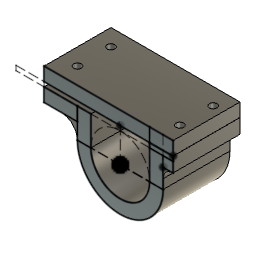
floorcowl_topfloor_edge v11 (Autodesk Fusion 360 design; units mm, degrees)
Autodesk Fusion 360 part; units mm, degrees
note: some values were not read from the file. Chosen so that the rebuilt part matches the saved one: which bodies a step acts on; which face or edge a step refers to.
sketch "Sketch1" plane through (0, 0, 0) normal (0, 1, 0) x (1, 0, 0)
  circle A0 centre (0, 0) radius 11.176 construction
  line L0 (0, 0) -> (0, -11.176) construction
  line L1 (0, -11.176) -> (0, -12.9286) construction
  line L2 (0, 0) -> (11.176, 0) construction
  line L3 (11.176, 0) -> (11.176, -11.176) construction
  line L4 (11.176, -11.176) -> (-39.624, -11.176) construction
  line L5 (-39.624, -11.176) -> (-39.624, -12.9286) construction
  line L6 (-39.624, -12.9286) -> (11.176, -12.9286) construction
  line L7 (11.176, -12.9286) -> (11.176, -11.176) construction
  line L8 (11.176, -12.9286) -> (-28.956, -12.9286)
  line L9 (-28.956, -12.9286) -> (-28.956, -18.0086)
  line L10 (-28.956, -18.0086) -> (11.176, -18.0086)
  line L11 (11.176, -18.0086) -> (11.176, -12.9286) construction
  line L12 (11.176, -18.0086) -> (16.256, -18.0086)
  line L13 (16.256, -18.0086) -> (16.256, 0)
  line L14 (16.256, 0) -> (11.176, 0)
  line L15 (11.176, 0) -> (11.176, -18.0086)
  arc A1 (16.256, 0) -> (-16.256, 0) centre (0, 0) ccw
  line L16 (0, 0) -> (16.256, 0) construction
  line L17 (0, 0) -> (-16.256, 0) construction
  arc A2 (11.176, 0) -> (-11.176, 0) centre (0, 0) ccw
  line L18 (0, 0) -> (11.176, 0) construction
  line L19 (0, 0) -> (-11.176, 0) construction
  line L20 (-11.176, 0) -> (-16.256, 0)
  line L21 (-16.256, 0) -> (-16.256, -11.176)
  line L22 (-16.256, -11.176) -> (-11.176, -11.176)
  line L23 (-11.176, -11.176) -> (-11.176, 0)
  line L24 (-16.256, -11.176) -> (-28.956, -11.176)
  line L25 (-28.956, -11.176) -> (-28.956, -6.096)
  line L26 (-28.956, -6.096) -> (-16.256, -6.096)
  line L27 (-16.256, -6.096) -> (-16.256, -11.176)
  line L28 (-28.956, -11.176) -> (-28.956, -12.9286) construction
  line L29 (16.256, -18.0086) -> (20.066, -18.0086)
  line L30 (20.066, -18.0086) -> (20.066, -12.9286)
  line L31 (11.176, -11.176) -> (16.256, -11.176)
  line L32 (16.256, -12.9286) -> (11.176, -12.9286) construction
  line L33 (20.066, -12.9286) -> (20.066, -11.176) construction
  line L34 (20.066, -11.176) -> (16.256, -11.176)
  line L35 (16.256, 0) -> (16.256, -11.176)
  line L36 (20.066, -11.176) -> (20.066, -7.366)
  line L37 (20.066, -7.366) -> (16.256, -7.366)
  line L38 (20.066, -12.9286) -> (11.176, -12.9286)
  line L39 (20.066, -11.176) -> (20.066, -12.8778)
  line L40 (20.066, -12.8778) -> (11.176, -12.8778)
  line L41 (11.176, -12.8778) -> (11.176, -11.176)
  line L42 (11.176, -11.176) -> (20.066, -11.176) construction
  line L43 (20.066, -11.176) -> (20.066, -12.8778)
  dimension "d1" = 22.352
  dimension "d2" = 1.7526
  dimension "d4" = 90
  dimension "d5" = 11.176
  dimension "d6" = 50.8
  dimension "d7" = 1.7526
  dimension "d9" = 5.08
  dimension "d10" = 5.08
  dimension "d11" = 18.0086
  dimension "d12" = 180
  dimension "d13" = 180
  dimension "d14" = 5.08
  dimension "d15" = 11.176
  dimension "d16" = 12.7
  dimension "d17" = 5.08
  dimension "d33" = 1.7526
  dimension "d42" = 3.81
  dimension "d43" = 5.08
  dimension "d44" = 1.7526
  dimension "d45" = 3.81
  dimension "d46" = 3.81
  dimension "d47" = 3.81
  dimension "d57" = 1.7018
  constraint coincident A0.centre L0.start
  constraint coincident A0 L0.end
  constraint vertical L0
  constraint parallel L0 L1
  constraint coincident A0 L2.end
  constraint perpendicular L0 L2
  constraint horizontal L4
  constraint vertical L5
  constraint horizontal L6
  constraint vertical L7
  constraint horizontal L8
  constraint vertical L9
  constraint horizontal L10
  constraint vertical L11
  constraint horizontal L12
  constraint vertical L13
  constraint horizontal L14
  constraint vertical L15
  constraint horizontal L20
  constraint vertical L21
  constraint horizontal L22
  constraint vertical L23
  constraint horizontal L24
  constraint vertical L25
  constraint horizontal L26
  constraint vertical L27
  constraint vertical L28
  constraint perpendicular L13 L29
  constraint perpendicular L29 L30
  constraint coincident L13 L32.start
  constraint coincident L13 L31.end
  constraint perpendicular L13 L31
  constraint horizontal L34
  constraint vertical L33
  constraint perpendicular L34 L36
  constraint perpendicular L13 L37
  constraint horizontal L32
  constraint perpendicular L34 L39
  constraint horizontal L40
  constraint vertical L41
  constraint horizontal L42
  constraint vertical L43
  measures "d1" diameter of A0
  measures "d2" distance of L0.end L1.end
  measures "d4" angle of L2 L3
  measures "d5" distance of L2.end L3.end
  measures "d6" distance of L3.end L4.end
  measures "d7" distance of L3.end L6.end
  measures "d9" distance of L6.end L10.end
  measures "d10" distance of L10.end L12.end
  measures "d11" distance of L12.end L13.end
  measures "d12" angle of L16 L17
  measures "d13" angle of L18 L19
  measures "d14" distance of A2.end A1.end
  measures "d15" distance of A2.end L22.end
  measures "d16" distance of L21.end L24.end
  measures "d17" distance of L21.end L26.end
  measures "d33" distance of L24.end L8.end
  measures "d42" distance of L12.end L29.end
  measures "d43" distance of L29.end L30.end
  measures "d44" distance of L30.end L33.end
  measures "d45" distance of L31.end L33.end
  measures "d46" distance of L33.end L36.end
  measures "d47" distance of L36.end L37.end
  measures "d57" distance of L33.end L39.end
extrude "Extrude1" add sketch "Sketch1" along normal blind 25.4 contours L8 L9 L10 L15 | L13 L14 L15 L31 L35 | L14 A1 A2 L20 | L20 L21 L22 L23 L27 | L21 L24 L25 L26 L27 makes body 1 at (-15.5787, 8.4667, 18.0086) makes body 2 at (-12.4528, 8.4667, -10.4492)
extrude "Extrude3" add sketch "Sketch1" along normal blind 25.4 contours L13 L15 L31 L40 L41 | L13 L34 L39 L40 L43 bodies 2
fillet "Fillet1" radius 6.35 1 edges at (-16.256, 12.7, 6.096) on bodies 2
sketch "Sketch4" plane through (0, 0, 18.0086) normal (0, 0, 1) x (-1, 0, 0)
  line L0 (28.956, 0) -> (-11.176, 0)
  line L1 (-11.176, -25.4) -> (28.956, -25.4)
  line L2 (28.956, -25.4) -> (28.956, 0)
  line L3 (28.956, -25.4) -> (16.256, -25.4)
  line L4 (16.256, -25.4) -> (16.256, 0)
  line L5 (16.256, 0) -> (28.956, 0)
  line L6 (28.956, 0) -> (28.956, -25.4)
  line L7 (28.956, -12.7) -> (16.256, -12.7)
  line L8 (22.606, -25.4) -> (22.606, 0)
  line L9 (-11.176, 0) -> (-11.176, -25.4)
  line L10 (-11.176, -25.4) -> (-16.256, -25.4) construction
  line L11 (-16.256, -25.4) -> (-16.256, 0) construction
  line L12 (-16.256, 0) -> (-11.176, 0) construction
  line L13 (16.256, -12.7) -> (-16.256, -12.7)
  point P0 (22.606, -19.05)
  point P1 (22.606, -6.35)
  point P2 (-16.256, -19.05)
  point P3 (-16.256, -6.35)
  dimension "d34" = 12.7
  dimension "d35" = 25.4
  dimension "d36" = 6.35
  dimension "d52" = 5.08
  dimension "d55" = 6.35
  dimension "d56" = 6.35
  constraint horizontal L3
  constraint vertical L4
  constraint horizontal L5
  constraint vertical L6
  constraint coincident L1.end L2.start
  constraint midpoint L2 L7.start
  constraint midpoint L4 L7.end
  constraint midpoint L3 L8.start
  constraint midpoint L5 L8.end
  constraint coincident L8 P0
  constraint symmetric L7 P0 P1
  constraint coincident L1.start L9.end
  constraint perpendicular L9 L10
  constraint perpendicular L10 L11
  constraint coincident L0.end L9.start
  constraint perpendicular L9 L12
  constraint midpoint L11 L13.end
  constraint coincident L11 P2
  constraint coincident L11 P3
  measures "d34" distance of L1.end L3.end
  measures "d35" distance of L1.end L0.start
  measures "d36" distance of L3 P0
  measures "d52" distance of L1.start L10.end
  measures "d55" distance of L10 P2
  measures "d56" distance of L11.end P3
extrude "Extrude2" add sketch "Sketch1" along normal blind 25.4 contours L12 L13 L15 L38 | L13 L29 L30 L38 | L13 L34 L35 L36 L37 bodies 2 1
fillet "Fillet2" radius 3.81 1 edges at (16.256, 12.7, 7.366) on bodies 2
hole "Hole4" at (16.256, 19.05, 18.0086) at (16.256, 6.35, 18.0086) direction (0, 0, -1) diameter 2.8702 depth 11.1125 tip angle 180 bodies 2 1
hole "Hole5" at (-22.606, 6.35, 18.0086) at (-22.606, 19.05, 18.0086) direction (0, 0, -1) diameter 2.8702 depth 10.16 tip angle 180 bodies 2 1
equation "d60 = ( 7 / 16 ) * 1 in"
